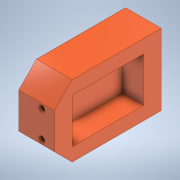
# Autodesk Inventor part: Print_Parts_Q
Saved by Autodesk Inventor 2020 (Build 240168000, 168)
## iProperties
Created: 2020-10-05
Part Number: Print_Parts_Q
Material: PC/ABS プラスチック
Document SubType Name: Modeling
Designer: kenta iguchi
Density: 0.357273 g/cm^3
Appearance: 滑らか - 淡いオレンジ
Author: kenta iguchi
Autodesk Inventor part; units mm, degrees
ref_plane "YZ Plane" through (0, 0, 0) normal (1, 0, 0) x (0, 1, 0)
ref_plane "XZ Plane" through (0, 0, 0) normal (0, 1, 0) x (-1, 0, 0)
ref_plane "XY Plane" through (0, 0, 0) normal (0, 0, 1) x (1, 0, 0)
sketch "スケッチ1" plane through (0, 0, 0) normal (0, 0, 1) x (1, 0, 0)
  line L0 (-10, -20) -> (10, -20)
  line L1 (10, -20) -> (10, 20)
  line L2 (10, 20) -> (-10, 20)
  line L3 (-10, 20) -> (-10, -20)
  line L4 (-10, -20) -> (10, 20) construction
  line L5 (10, -20) -> (-10, 20) construction
  point P0 (0, 0)
  dimension "d0" = 20
  dimension "d1" = 40
  constraints: 12 end point, 2 midpoint, 2 parallel, 1 horizontal, 1 perpendicular
  measures "d0" distance of L2.end L1.end
  measures "d1" distance of L1.end L0.end
extrude "押し出し1" add sketch "スケッチ1" along normal blind 10
sketch "スケッチ2" plane through (0, 0, 10) normal (0, 0, 1) x (1, 0, 0)
  line L0 (-10, 20) -> (-10, -20) projected
  line L1 (-10, -20) -> (10, -20) projected
  line L2 (10, -20) -> (10, 20) projected
  line L3 (10, 20) -> (-10, 20) projected
  line L4 (10, 20) -> (-10, 20)
  line L5 (-10, 20) -> (-10, 12.5)
  line L6 (-10, 12.5) -> (10, 12.5)
  line L7 (10, 12.5) -> (10, 20)
  line L8 (10, -20) -> (-10, -20)
  line L9 (-10, -20) -> (-10, -12.5)
  line L10 (-10, -12.5) -> (10, -12.5)
  line L11 (10, -12.5) -> (10, -20)
  line L12 (-10, 20) -> (-2, 20)
  line L13 (-2, 20) -> (-2, -20)
  line L14 (-2, -20) -> (-10, -20)
  line L15 (-10, -20) -> (-10, 20)
  point P0 (0, 0)
  point P1 (10, -12.5)
  point P2 (-2, -12.5)
  point P3 (-2, 12.5)
  point P4 (10, 12.5)
  dimension "d4" = 7.5
  dimension "d5" = 7.5
  dimension "d6" = 8
  constraints: 24 end point, 6 parallel, 3 horizontal, 3 perpendicular, 2 point on line, 1 vertical alignment
  measures "d4" distance between parallel lines of L3 L6
  measures "d5" distance between parallel lines of L1 L10
  measures "d6" distance between parallel lines of L13 L0
extrude "押し出し2" add sketch "スケッチ2" along normal blind 40 contours L3 L13 L6 L0 | L6 L13 L10 L0 | L3 L2 L6 L13 | L10 L13 L1 L0 | L10 L2 L1 L13
sketch "スケッチ3" plane through (0, 0, 50) normal (0, 0, 1) x (1, 0, 0)
  line L0 (-10, -20) -> (10, -20) projected
  line L1 (10, -20) -> (10, -12.5) projected
  line L2 (10, 12.5) -> (10, 20) projected
  line L3 (10, 20) -> (-10, 20) projected
  line L4 (-10, 20) -> (-10, -20) projected
  line L5 (10, 12.5) -> (-2, 12.5) projected
  line L6 (-2, 12.5) -> (-2, -12.5) projected
  line L7 (-2, -12.5) -> (10, -12.5) projected
  line L8 (10, -12.5) -> (10, 12.5) projected
  point P0 (0, 0)
extrude "押し出し3" add sketch "スケッチ3" along normal blind 10
sketch "スケッチ4" plane through (0, 0, 60) normal (0, 0, 1) x (1, 0, 0)
  line L0 (10, -20) -> (10, 20) projected
  point P0 (0, 0)
  point P1 (3, 7.5)
  point P2 (3, -7.5)
  dimension "d11" = 7
  dimension "d12" = 15
  dimension "d13" = 7.5
  constraints: 1 vertical alignment
  measures "d11" distance from line of L0 point (3, 7.5)
  measures "d12" distance of point (3, 7.5) point (3, -7.5)
  measures "d13" vertical distance of point (0, 0) point (3, 7.5)
hole "穴1" at (3, 7.5, 60) at (3, -7.5, 60) direction (0, 0, -1) diameter 3.3 depth 40.25
chamfer "面取り1" distance 10 angle 45 2 edges at (0, 20, 60) (0, -20, 60)
